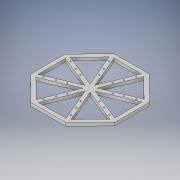
# Autodesk Inventor part: BODYFINAL
Saved by Autodesk Inventor 2018 (Build 220112000, 112)
## iProperties
Created: 2018-01-08
Part Number: BODYFINAL
Material: Generic
Document SubType Name: Modeling
Designer: BB-8
Density: 1 g/cm^3
Appearance: Default
Author: BB-8
Autodesk Inventor part; units mm, degrees
ref_plane "YZ Plane" through (0, 0, 0) normal (1, 0, 0) x (0, 1, 0)
ref_plane "XZ Plane" through (0, 0, 0) normal (0, 1, 0) x (-1, 0, 0)
ref_plane "XY Plane" through (0, 0, 0) normal (0, 0, 1) x (1, 0, 0)
sketch "Sketch3" plane through (0, 0, 0) normal (0, 1, 0) x (-1, 0, 0)
  line L0 (28.0459, -66.2904) -> (-27.0429, -66.7058)
  line L1 (-27.0429, -66.7058) -> (-66.2904, -28.0459)
  line L2 (-66.2904, -28.0459) -> (-66.7058, 27.0429)
  line L3 (-66.7058, 27.0429) -> (-28.0459, 66.2904)
  line L4 (-28.0459, 66.2904) -> (27.0429, 66.7058)
  line L5 (27.0429, 66.7058) -> (66.2904, 28.0459)
  line L6 (66.2904, 28.0459) -> (66.7058, -27.0429)
  line L7 (66.7058, -27.0429) -> (28.0459, -66.2904)
  line L8 (60.6628, -21.3559) -> (60.3338, 22.2684)
  line L9 (57.9959, 27.7942) -> (26.9163, 58.4085)
  line L10 (21.3559, 60.6628) -> (-22.2684, 60.3338)
  line L11 (-27.7942, 57.9959) -> (-58.4085, 26.9163)
  line L12 (-60.6628, 21.3559) -> (-60.3338, -22.2684)
  line L13 (-57.9959, -27.7942) -> (-26.9163, -58.4085)
  line L14 (-21.3559, -60.6628) -> (22.2684, -60.3338)
  line L15 (27.7942, -57.9959) -> (58.4085, -26.9163)
  circle A0 centre (21.4203, 52.1128) radius 1
  circle A1 centre (15.3792, 37.9354) radius 1
  circle A2 centre (10.3932, 25.6366) radius 1
  circle A3 centre (-21.7028, 51.9958) radius 1
  circle A4 centre (-15.9496, 37.6991) radius 1
  circle A5 centre (-10.7787, 25.4769) radius 1
  circle A6 centre (-52.1128, 21.4203) radius 1
  circle A7 centre (-37.9354, 15.3792) radius 1
  circle A8 centre (-25.6366, 10.3932) radius 1
  circle A9 centre (-51.9958, -21.7028) radius 1
  circle A10 centre (-37.6991, -15.9496) radius 1
  circle A11 centre (-25.4769, -10.7787) radius 1
  circle A12 centre (-21.4203, -52.1128) radius 1
  circle A13 centre (-15.3792, -37.9354) radius 1
  circle A14 centre (-10.3932, -25.6366) radius 1
  circle A15 centre (21.7028, -51.9958) radius 1
  circle A16 centre (15.9496, -37.6991) radius 1
  circle A17 centre (10.7787, -25.4769) radius 1
  circle A18 centre (52.1128, -21.4203) radius 1
  circle A19 centre (37.9354, -15.3792) radius 1
  circle A20 centre (25.6366, -10.3932) radius 1
  circle A21 centre (51.9958, 21.7028) radius 1
  circle A22 centre (37.6991, 15.9496) radius 1
  circle A23 centre (25.4769, 10.7787) radius 1
  line L16 (60.6628, -21.3559) -> (7.8392, 0.0591)
  line L17 (-5.5849, 5.5013) -> (-58.4085, 26.9163)
  line L18 (-22.2684, 60.3338) -> (-0.0591, 7.8392)
  line L19 (5.5849, -5.5013) -> (27.7942, -57.9959)
  line L20 (26.9163, 58.4085) -> (5.5013, 5.5849)
  line L21 (0.0591, -7.8392) -> (-21.3559, -60.6628)
  line L22 (60.3338, 22.2684) -> (7.8392, 0.0591)
  line L23 (-5.5013, -5.5849) -> (-57.9959, -27.7942)
  line L24 (58.4085, -26.9163) -> (5.5849, -5.5013)
  line L25 (-7.8392, -0.0591) -> (-60.6628, 21.3559)
  line L26 (57.9959, 27.7942) -> (5.5013, 5.5849)
  line L27 (-7.8392, -0.0591) -> (-60.3338, -22.2684)
  line L28 (-27.7942, 57.9959) -> (-5.5849, 5.5013)
  line L29 (0.0591, -7.8392) -> (22.2684, -60.3338)
  line L30 (21.3559, 60.6628) -> (-0.0591, 7.8392)
  line L31 (-5.5013, -5.5849) -> (-26.9163, -58.4085)
  point P0 (0, 0)
  point P1 (0, 0)
  dimension "d4" = 133
  dimension "d5" = 133
  dimension "d6" = 6
  dimension "d15" = 2
  dimension "d16" = 2
  dimension "d17" = 2
  dimension "d20" = 360
  dimension "d22" = 13.4108
  dimension "d23" = 11.271
  constraints: 64 end point, 24 centre point, 1 coincident, 66 other
  measures "d4" distance between parallel lines of L2 L6
  measures "d5" distance between parallel lines of L4 L0
  measures "d6" distance between parallel lines of L6 L8
  measures "d15" diameter of A0
  measures "d16" diameter of A1
  measures "d17" diameter of A2
extrude "Extrusion2" add sketch "Sketch3" along normal blind 5
body "Solid2"
